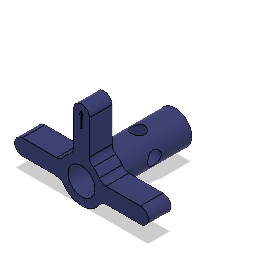
3way_knob_existing v16 (Autodesk Fusion 360 design; units mm, degrees)
Autodesk Fusion 360 part; units mm, degrees
sketch "Sketch1" plane through (0, 0, 0) normal (0, 0, 1) x (1, 0, 0)
  circle A0 centre (0, 0) radius 3.175
  dimension "d1" = 6.35
  measures "d1" diameter of A0
extrude "Extrude1" add sketch "Sketch1" along normal blind 10.668 and the other way blind 7.112 makes body 1
sketch "Sketch2" plane through (0, 0, 10.668) normal (0, 0, 1) x (1, 0, 0)
  circle A0 centre (0, 0) radius 3.175
  line L0 (-1.524, 3.7674) -> (-1.524, 12.7)
  line L1 (1.524, 3.7674) -> (1.524, 12.7)
  line L2 (1.524, 12.7) -> (-1.524, 12.7)
  line L3 (-3.7674, 1.524) -> (-12.7, 1.524)
  line L4 (-12.7, 1.524) -> (-12.7, -1.524)
  line L5 (-12.7, -1.524) -> (-3.7674, -1.524)
  arc A1 (-1.524, 3.7674) -> (-3.7674, 1.524) centre (0, 0) ccw
  line L6 (0, -6.858) -> (0, 16.002) construction
  line L7 (3.7674, 1.524) -> (12.7, 1.524)
  line L8 (12.7, 1.524) -> (12.7, -1.524)
  line L9 (12.7, -1.524) -> (3.7674, -1.524)
  arc A2 (-3.7674, -1.524) -> (3.7674, -1.524) centre (0, 0) ccw
  arc A3 (3.7674, 1.524) -> (1.524, 3.7674) centre (0, 0) ccw
  dimension "d6" = 8.128
  dimension "d7" = 3.048
  dimension "d8" = 1.524
  dimension "d9" = 12.7
  dimension "d10" = 12.7
  dimension "d11" = 1.524
  dimension "d12" = 3.048
  dimension "d14" = 1.524
  dimension "d15" = 3.048
  measures "d6" diameter of A1
  measures "d7" distance of L0 L1
  measures "d8" distance of A0.centre L0
  measures "d9" distance of A0.centre L2
  measures "d10" distance of L4 A0.centre
  measures "d11" distance of L5 A0.centre
  measures "d12" distance of L3 L5
  measures "d14" distance of L7 A0.centre
  measures "d15" distance of L7 L9
extrude "Extrude2" add sketch "Sketch2" against normal blind 4.318 bodies 1
sketch "Sketch3" plane through (0, 0, 10.668) normal (0, 0, 1) x (1, 0, 0)
  line L0 (12.7, 1.524) -> (3.7674, 1.524)
  arc A0 (3.7674, 1.524) -> (1.524, 3.7674) centre (0, 0) ccw
  line L1 (1.524, 3.7674) -> (1.524, 12.7)
  line L2 (1.524, 12.7) -> (-1.524, 12.7)
  line L3 (-1.524, 12.7) -> (-1.524, 3.7674)
  arc A1 (-1.524, 3.7674) -> (-3.7674, 1.524) centre (0, 0) ccw
  line L4 (-3.7674, 1.524) -> (-12.7, 1.524)
  line L5 (-12.7, 1.524) -> (-12.7, -1.524)
  line L6 (-12.7, -1.524) -> (-3.7674, -1.524)
  arc A2 (-3.7674, -1.524) -> (3.7674, -1.524) centre (0, 0) ccw
  line L7 (3.7674, -1.524) -> (12.7, -1.524)
  line L8 (12.7, -1.524) -> (12.7, 1.524)
  circle A3 centre (0, 0) radius 3.175 construction
  line L9 (-3.175, 0) -> (3.175, 0)
  point P0 (-3.175, 0)
sketch "Sketch4" plane through (0, 0, 10.668) normal (0, 0, 1) x (1, 0, 0)
  circle A0 centre (0, 0) radius 2.54
  dimension "d18" = 5.08
  measures "d18" diameter of A0
extrude "Extrude3" cut sketch "Sketch4" against normal blind 25.4 bodies 1
sketch "Sketch5" plane through (0, 0, 0) normal (1, 0, 0) x (0, 0, -1)
  line L0 (0, 0) -> (0, 3.175)
  dimension "d21" = 3.175
  measures "d21" distance of L0.start L0.end
fillet "Fillet1" radius 1.524 6 edges at (-1.524, 12.7, 8.509) (1.524, 12.7, 8.509) (12.7, 1.524, 8.509) (-12.7, 1.524, 8.509) (-12.7, -1.524, 8.509) (12.7, -1.524, 8.509) on bodies 1
fillet "Fillet2" radius 1.524 6 edges at (-3.7674, -1.524, 8.509) (3.7674, -1.524, 8.509) (3.7674, 1.524, 8.509) (1.524, 3.7674, 8.509) (-1.524, 3.7674, 8.509) (-3.7674, 1.524, 8.509) on bodies 1
sketch "Sketch6" plane through (0, 0, 0) normal (0, 0, 1) x (1, 0, 0)
  line L0 (-3.175, 0) -> (3.175, 0)
  circle A0 centre (0, 0) radius 3.175 construction
  circle A1 centre (0, 0) radius 3.175
sketch "Sketch10" plane through (0, 0, 0) normal (0, 0, 1) x (1, 0, 0)
sketch "Sketch11" plane through (0, 0, 0) normal (1, 0, 0) x (0, 0, -1)
  circle A0 centre (0, 0) radius 1.778
  dimension "d46" = 3.556
  measures "d46" diameter of A0
extrude "Extrude7" add sketch "Sketch11" along normal blind 3.175 and the other way blind 3.175 separate body makes body 2
sketch "Sketch12" plane through (0, 0, 0) normal (0, 1, 0) x (1, 0, 0)
  circle A0 centre (0, 0) radius 1.778
  dimension "d51" = 3.556
  measures "d51" diameter of A0
extrude "Extrude8" add sketch "Sketch12" along normal blind 3.175 separate body makes body 3
combine "Combine1" operation add target body 3 tool bodies 2
fillet "Fillet6" radius 0.127 2 edges at (1.778, 1.778, 0) (-1.778, 1.778, 0) on bodies 3
combine "Combine2" operation add target body 1 tool bodies 3
sketch "Sketch13" plane through (0, 3.175, 0) normal (0, 1, 0) x (-1, 0, 0)
  circle A0 centre (0, 0) radius 1.778
  circle A1 centre (0, 0) radius 1.27
  dimension "d55" = 2.54
  measures "d55" diameter of A1
extrude "Extrude9" cut sketch "Sketch13" against normal blind 3.175 contours A1 bodies 1
sketch "Sketch14" plane through (3.175, 0, 0) normal (1, 0, 0) x (0, 0, -1)
  circle A0 centre (0, 0) radius 1.778
  circle A1 centre (0, 0) radius 1.27
  dimension "d58" = 2.54
  measures "d58" diameter of A1
extrude "Extrude10" cut sketch "Sketch14" against normal blind 16.764 contours A1 bodies 1
fillet "Fillet7" radius 0.0762 2 edges at (-1.27, 1.27, 0) (1.27, 1.27, 0) on bodies 1
sketch "Sketch15" plane through (0, 0, -7.112) normal (0, 0, -1) x (-1, 0, 0)
  circle A0 centre (0, 0) radius 2.54
  circle A1 centre (0, 0) radius 3.175
  circle A2 centre (0, 0) radius 3.175
  circle A3 centre (0, 0) radius 6.35
  dimension "d62" = 6.35
  dimension "d63" = 12.7
  measures "d62" diameter of A2
  measures "d63" diameter of A3
extrude "Extrude11" cut sketch "Sketch15" against normal blind 10.16 contours A3 bodies 1
sketch "Sketch16" plane through (0, 0, 10.668) normal (0, 0, 1) x (1, 0, 0)
  circle A0 centre (0, 0) radius 2.54
  arc A1 (11.176, -1.524) -> (11.176, 1.524) centre (11.176, 0) ccw
  line L0 (11.176, 1.524) -> (4.6835, 1.524)
  arc A2 (3.4062, 2.2167) -> (4.6835, 1.524) centre (4.6835, 3.048) ccw
  arc A3 (3.4062, 2.2167) -> (2.2167, 3.4062) centre (0, 0) ccw
  arc A4 (1.524, 4.6835) -> (2.2167, 3.4062) centre (3.048, 4.6835) ccw
  line L1 (1.524, 4.6835) -> (1.524, 11.176)
  arc A5 (1.524, 11.176) -> (-1.524, 11.176) centre (0, 11.176) ccw
  line L2 (-1.524, 11.176) -> (-1.524, 4.6835)
  arc A6 (-2.2167, 3.4062) -> (-1.524, 4.6835) centre (-3.048, 4.6835) ccw
  arc A7 (-2.2167, 3.4062) -> (-3.4062, 2.2167) centre (0, 0) ccw
  arc A8 (-4.6835, 1.524) -> (-3.4062, 2.2167) centre (-4.6835, 3.048) ccw
  line L3 (-4.6835, 1.524) -> (-11.176, 1.524)
  arc A9 (-11.176, 1.524) -> (-11.176, -1.524) centre (-11.176, 0) ccw
  line L4 (-11.176, -1.524) -> (-4.6835, -1.524)
  arc A10 (-3.4062, -2.2167) -> (-4.6835, -1.524) centre (-4.6835, -3.048) ccw
  arc A11 (-3.4062, -2.2167) -> (3.4062, -2.2167) centre (0, 0) ccw
  arc A12 (4.6835, -1.524) -> (3.4062, -2.2167) centre (4.6835, -3.048) ccw
  line L5 (4.6835, -1.524) -> (11.176, -1.524)
  line L6 (-0.254, 10.922) -> (0, 11.557)
  line L7 (0, 11.557) -> (0.254, 10.922)
  line L8 (0.254, 10.922) -> (0.127, 10.922)
  line L9 (0.127, 10.922) -> (0.127, 8.7121)
  line L10 (0.127, 8.7121) -> (-0.127, 8.7121)
  line L11 (-0.127, 8.7121) -> (-0.127, 10.922)
  line L12 (-0.127, 10.922) -> (-0.254, 10.922)
extrude "Extrude12" add sketch "Sketch16" along normal blind 0.127 contours L6 L7 L8 L9 L10 L11 L12 bodies 1
equation "d6 = 0.2 in + 0.12 in"
equation "d9 = 0.34 in + 0.16 in"
